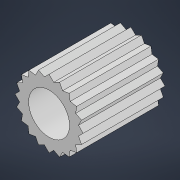
# Autodesk Inventor part: fancy spacer
Saved by Autodesk Inventor 2022 (Build 260153000, 153)
## iProperties
Created: 2022-02-08
Part Number: fancy spacer
Material: Generic
Document SubType Name: Modeling
Designer: nicol
Density: 1 g/cm^3
Appearance: Default
Author: nicol
Autodesk Inventor part; units mm, degrees
ref_plane "YZ Plane" through (0, 0, 0) normal (1, 0, 0) x (0, 1, 0)
ref_plane "XZ Plane" through (0, 0, 0) normal (0, 1, 0) x (-1, 0, 0)
ref_plane "XY Plane" through (0, 0, 0) normal (0, 0, 1) x (1, 0, 0)
sketch "Sketch1" plane through (0, 0, 0) normal (0, 0, 1) x (1, 0, 0)
  circle A0 centre (0, 0) radius 1.5
  circle A1 centre (0, 0) radius 2.5 construction
  circle A2 centre (0, 0) radius 1.9
  line L0 (-0.7576, 1.7424) -> (0, 2.5)
  line L1 (0, 2.5) -> (0.7576, 1.7424)
  line L2 (0, 2.5) -> (0, 0) construction
  line L3 (-1.2589, 1.4231) -> (-0.7725, 2.3776)
  line L4 (-0.7725, 2.3776) -> (0.182, 1.8913)
  line L5 (-1.6371, 0.9644) -> (-1.4695, 2.0225)
  line L6 (-1.4695, 2.0225) -> (-0.4113, 1.8549)
  line L7 (-1.8549, 0.4113) -> (-2.0225, 1.4695)
  line L8 (-2.0225, 1.4695) -> (-0.9644, 1.6371)
  line L9 (-1.8913, -0.182) -> (-2.3776, 0.7725)
  line L10 (-2.3776, 0.7725) -> (-1.4231, 1.2589)
  line L11 (-1.7424, -0.7576) -> (-2.5, 0)
  line L12 (-2.5, 0) -> (-1.7424, 0.7576)
  line L13 (-1.4231, -1.2589) -> (-2.3776, -0.7725)
  line L14 (-2.3776, -0.7725) -> (-1.8913, 0.182)
  line L15 (-0.9644, -1.6371) -> (-2.0225, -1.4695)
  line L16 (-2.0225, -1.4695) -> (-1.8549, -0.4113)
  line L17 (-0.4113, -1.8549) -> (-1.4695, -2.0225)
  line L18 (-1.4695, -2.0225) -> (-1.6371, -0.9644)
  line L19 (0.182, -1.8913) -> (-0.7725, -2.3776)
  line L20 (-0.7725, -2.3776) -> (-1.2589, -1.4231)
  line L21 (0.7576, -1.7424) -> (0, -2.5)
  line L22 (0, -2.5) -> (-0.7576, -1.7424)
  line L23 (1.2589, -1.4231) -> (0.7725, -2.3776)
  line L24 (0.7725, -2.3776) -> (-0.182, -1.8913)
  line L25 (1.6371, -0.9644) -> (1.4695, -2.0225)
  line L26 (1.4695, -2.0225) -> (0.4113, -1.8549)
  line L27 (1.8549, -0.4113) -> (2.0225, -1.4695)
  line L28 (2.0225, -1.4695) -> (0.9644, -1.6371)
  line L29 (1.8913, 0.182) -> (2.3776, -0.7725)
  line L30 (2.3776, -0.7725) -> (1.4231, -1.2589)
  line L31 (1.7424, 0.7576) -> (2.5, 0)
  line L32 (2.5, 0) -> (1.7424, -0.7576)
  line L33 (1.4231, 1.2589) -> (2.3776, 0.7725)
  line L34 (2.3776, 0.7725) -> (1.8913, -0.182)
  line L35 (0.9644, 1.6371) -> (2.0225, 1.4695)
  line L36 (2.0225, 1.4695) -> (1.8549, 0.4113)
  line L37 (0.4113, 1.8549) -> (1.4695, 2.0225)
  line L38 (1.4695, 2.0225) -> (1.6371, 0.9644)
  line L39 (-0.182, 1.8913) -> (0.7725, 2.3776)
  line L40 (0.7725, 2.3776) -> (1.2589, 1.4231)
  point P0 (-0.992, 1.9469)
  point P1 (-1.5451, 1.5451)
  point P2 (-1.9469, 0.992)
  point P3 (-2.1582, 0.3418)
  point P4 (-2.1582, -0.3418)
  point P5 (-1.9469, -0.992)
  point P6 (-1.5451, -1.5451)
  point P7 (-0.992, -1.9469)
  point P8 (-0.3418, -2.1582)
  point P9 (0.3418, -2.1582)
  point P10 (0.992, -1.9469)
  point P11 (1.5451, -1.5451)
  point P12 (1.9469, -0.992)
  point P13 (2.1582, -0.3418)
  point P14 (2.1582, 0.3418)
  point P15 (1.9469, 0.992)
  point P16 (1.5451, 1.5451)
  point P17 (0.992, 1.9469)
  point P18 (0.3418, 2.1582)
  point P19 (-0.3418, 2.1582)
  dimension "d1" = 5
  dimension "d0" = 3
  dimension "d2" = 0.4
  dimension "d5" = 360
  constraints: 82 end point, 2 centre point, 2 coincident, 2 perpendicular, 2 point on circle, 1 vertical, 1 vertical alignment, 103 other
  measures "d0" diameter of A0
  measures "d2" radial gap between concentric circles of A0 A2
extrude "Extrusion1" add sketch "Sketch1" along normal blind 6
body "Solid1"
